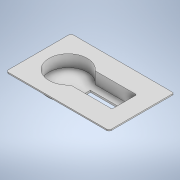
# Autodesk Inventor part: badge
Saved by Autodesk Inventor 2020 (Build 240168000, 168)
## iProperties
Created: 2019-12-22
Part Number: badge
Material: Generic
Document SubType Name: Modeling
Designer: user
Density: 1 g/cm^3
Appearance: Default
Author: user
## iProperties of the stored document _3DPrint.ipt
Created: 2019-12-23
Part Number: _3DPrint
Material: Generic
Document SubType Name: Modeling
Designer: user
Density: 1 g/cm^3
Appearance: Default
Author: user
Autodesk Inventor part; units mm, degrees
ref_plane "YZ Plane" through (0, 0, 0) normal (1, 0, 0) x (0, 1, 0)
ref_plane "XZ Plane" through (0, 0, 0) normal (0, 1, 0) x (-1, 0, 0)
ref_plane "XY Plane" through (0, 0, 0) normal (0, 0, 1) x (1, 0, 0)
sketch "Sketch1" plane through (0, 0, 0) normal (0, 1, 0) x (-1, 0, 0)
  circle A0 centre (-14.0224, -4.7987) radius 17
  line L0 (-61.8084, 4.4628) -> (-61.8084, -14.0372)
  line L1 (-59.8084, -16.0372) -> (-26.7776, -16.0372)
  line L2 (-26.7573, 6.4628) -> (-59.8084, 6.4628)
  arc A1 (-61.8084, -14.0372) -> (-59.8084, -16.0372) centre (-59.8084, -14.0372) ccw
  arc A2 (-59.8084, 6.4628) -> (-61.8084, 4.4628) centre (-59.8084, 4.4628) ccw
  line L3 (-28.2727, -0.5372) -> (-54.8084, -0.5372)
  line L4 (-54.8084, -0.5372) -> (-54.8084, -9.0372)
  line L5 (-54.8084, -9.0372) -> (-28.2727, -9.0372)
  line L6 (-28.2727, -9.0372) -> (-28.2727, -0.5372)
  line L7 (8.6213, 22.2028) -> (-72.9787, 22.2028)
  line L8 (-73.8987, -31.7772) -> (8.6213, -31.7772)
  line L9 (10.6213, -29.7772) -> (10.6213, 20.2028)
  line L10 (-74.9787, 20.2028) -> (-74.9787, 4.3773)
  line L11 (-74.9787, -30.6972) -> (-74.9787, -14.8717)
  arc A3 (-74.9787, -30.6972) -> (-73.8987, -31.7772) centre (-73.8987, -30.6972) ccw
  arc A4 (-72.9787, 22.2028) -> (-74.9787, 20.2028) centre (-72.9787, 20.2028) ccw
  arc A5 (10.6213, 20.2028) -> (8.6213, 22.2028) centre (8.6213, 20.2028) ccw
  arc A6 (8.6213, -31.7772) -> (10.6213, -29.7772) centre (8.6213, -29.7772) ccw
  line L12 (-74.9787, 4.3773) -> (-74.9787, -14.8717)
  circle A7 centre (-14.0224, -4.7987) radius 16
  line L13 (-27.4955, -15.0372) -> (-59.8084, -15.0372)
  line L14 (-60.8084, -14.0372) -> (-60.8084, 4.4628)
  arc A8 (-60.8084, -14.0372) -> (-59.8084, -15.0372) centre (-59.8084, -14.0372) ccw
  line L15 (-59.8084, 5.4628) -> (-27.576, 5.4628)
  arc A9 (-59.8084, 5.4628) -> (-60.8084, 4.4628) centre (-59.8084, 4.4628) ccw
  line L16 (-26.7776, -16.0372) -> (-25.4108, -16.0372)
  line L17 (-27.4955, -15.0372) -> (-26.3176, -15.0372)
  line L18 (-27.576, 5.4628) -> (-26.2984, 5.4628)
  line L19 (-26.7573, 6.4628) -> (-25.388, 6.4628)
  point P0 (0, 0)
  point P1 (-61.8084, -16.0372)
  dimension "d20" = 34
  dimension "d26" = 2
  dimension "d28" = 7
  dimension "d32" = 7
  dimension "d167" = 8.5
  dimension "d171" = 26.5357
  dimension "d177" = 85.6
  dimension "d229" = 32
  dimension "d230" = 1
  dimension "d231" = 1
  dimension "d232" = 1
  dimension "d233" = 1
  dimension "d234" = 1
  dimension "d235" = 1
  dimension "d241" = 53.98
  dimension "d242" = 22.74
  dimension "d243" = 22.74
  dimension "d248" = 62.786
  dimension "d249" = 6
  constraints: 40 end point, 23 point on circle, 16 tangent, 10 centre point, 6 horizontal, 6 parallel, 3 perpendicular, 3 point on line, 3 vertical, 2 equal radius
  measures "d20" diameter of A0
  measures "d26" radius of A1
  measures "d28" distance between parallel lines of L1 L5
  measures "d32" distance between parallel lines of L3 L2
  measures "d167" distance between parallel lines of L3 L5
  measures "d171" distance between parallel lines of L4 L6
  measures "d177" distance between parallel lines of L11 L9
  measures "d229" diameter of A7
  measures "d230" radial gap between concentric circles of A0 A7
  measures "d231" distance between parallel lines of L13 L1
  measures "d232" distance between parallel lines of L0 L14
  measures "d233" radius of A8
  measures "d234" distance between parallel lines of L2 L15
  measures "d235" radius of A9
  measures "d241" distance between parallel lines of L8 L7
  measures "d242" distance between parallel lines of L8 L5
  measures "d243" distance between parallel lines of L7 L3
  measures "d249" distance between parallel lines of L4 L14
extrude "Extrusion22" add sketch "Sketch1" along normal blind 1
extrude "Extrusion23" add sketch "Sketch1" against normal blind 10.5 contours A0 L16 A7 L19 | L19 A7 L18 A0 | A0 L15 A9 L14 A8 L13 L1 A1 L0 A2 L2 | A0 L13 L17 A7 L16 | L18 A7 L3 A0 | A0 L3 L4 L5 L13 A8 L14 A9 L15 | A7 L5 L6 L3 | A0 L5 A7 L17 L13 picked at (-18.1893, -4.791)
extrude "Extrusion24" cut sketch "Sketch1" against normal blind 9 contours L18 A7 L3 A0 | A0 L3 L4 L5 L13 A8 L14 A9 L15 | A7 L5 L6 L3 | A0 L5 A7 L17 L13 picked at (-18.1893, -4.791)
extrude "Extrusion25" add sketch "Sketch1" along normal blind 1 contours A0 L16 A7 L19 | L19 A7 L18 A0 | A0 L15 A9 L14 A8 L13 L1 A1 L0 A2 L2 | A0 L13 L17 A7 L16
sketch "Sketch24" plane through (0, 0, 0) normal (0, -1, 0) x (1, 0, 0)
  line L0 (30.3846, -19.8888) -> (77.1521, -19.8888) construction
  line L1 (77.1521, -19.8888) -> (77.1521, -30.5341) construction
  line L2 (77.1521, -30.5341) -> (30.3846, -30.5341) construction
  line L3 (30.3846, -30.5341) -> (30.3846, -19.8888) construction
  line L4 (40.073, -25.6301) -> (61.0048, -25.6301) construction
  line L5 (61.0048, -25.6301) -> (61.0048, -28.2616) construction
  line L6 (61.0048, -28.2616) -> (40.073, -28.2616) construction
  line L7 (40.073, -28.2616) -> (40.073, -25.6301) construction
  spline S0 degree 2 poles (31.7579, -23.0554) (31.4887, -23.0554) (31.0885, -22.9146) (30.9477, -22.7738) knots 0 0 0 1 2 2 2
  spline S1 degree 2 poles (30.9477, -22.7738) (30.7872, -22.6157) (30.6563, -22.1711) (30.6563, -21.8451) knots 0 0 0 1 2 2 2
  line L8 (30.6563, -21.8451) -> (30.6563, -19.9432)
  line L9 (30.6563, -19.9432) -> (31.0614, -19.9432)
  line L10 (31.0614, -19.9432) -> (31.0614, -21.8451)
  spline S2 degree 2 poles (31.0614, -21.8451) (31.0614, -22.0575) (31.1157, -22.344) (31.1923, -22.4601) knots 0 0 0 1 2 2 2
  spline S3 degree 2 poles (31.1923, -22.4601) (31.2738, -22.5836) (31.5554, -22.7096) (31.7579, -22.7096) knots 0 0 0 1 2 2 2
  spline S4 degree 2 poles (31.7579, -22.7096) (31.9481, -22.7096) (32.2445, -22.5836) (32.326, -22.4601) knots 0 0 0 1 2 2 2
  spline S5 degree 2 poles (32.326, -22.4601) (32.4026, -22.344) (32.4569, -22.06) (32.4569, -21.855) knots 0 0 0 1 2 2 2
  line L11 (32.4569, -21.855) -> (32.4569, -19.9432)
  line L12 (32.4569, -19.9432) -> (32.862, -19.9432)
  line L13 (32.862, -19.9432) -> (32.862, -21.8451)
  spline S6 degree 2 poles (32.862, -21.8451) (32.862, -22.1637) (32.7336, -22.6182) (32.5705, -22.7738) knots 0 0 0 1 2 2 2
  spline S7 degree 2 poles (32.5705, -22.7738) (32.4248, -22.9171) (32.0395, -23.0554) (31.7579, -23.0554) knots 0 0 0 1 2 2 2
  line L14 (35.6655, -22.9912) -> (35.1393, -22.9912)
  line L15 (35.1393, -22.9912) -> (34.0254, -21.5734)
  line L16 (34.0254, -21.5734) -> (33.8475, -21.7735)
  line L17 (33.8475, -21.7735) -> (33.8475, -22.9912)
  line L18 (33.8475, -22.9912) -> (33.4424, -22.9912)
  line L19 (33.4424, -22.9912) -> (33.4424, -19.9432)
  line L20 (33.4424, -19.9432) -> (33.8475, -19.9432)
  line L21 (33.8475, -19.9432) -> (33.8475, -21.3437)
  line L22 (33.8475, -21.3437) -> (35.0974, -19.9432)
  line L23 (35.0974, -19.9432) -> (35.5914, -19.9432)
  line L24 (35.5914, -19.9432) -> (34.3292, -21.3042)
  line L25 (34.3292, -21.3042) -> (35.6655, -22.9912)
  line L26 (38.2787, -22.9912) -> (37.0981, -22.9912)
  line L27 (37.0981, -22.9912) -> (37.0981, -22.68)
  line L28 (37.0981, -22.68) -> (37.4859, -22.68)
  line L29 (37.4859, -22.68) -> (37.4859, -20.2544)
  line L30 (37.4859, -20.2544) -> (37.0981, -20.2544)
  line L31 (37.0981, -20.2544) -> (37.0981, -19.9432)
  line L32 (37.0981, -19.9432) -> (38.2787, -19.9432)
  line L33 (38.2787, -19.9432) -> (38.2787, -20.2544)
  line L34 (38.2787, -20.2544) -> (37.8909, -20.2544)
  line L35 (37.8909, -20.2544) -> (37.8909, -22.68)
  line L36 (37.8909, -22.68) -> (38.2787, -22.68)
  line L37 (38.2787, -22.68) -> (38.2787, -22.9912)
  line L38 (40.9612, -22.9912) -> (40.5067, -22.9912)
  line L39 (40.5067, -22.9912) -> (39.1581, -20.3631)
  line L40 (39.1581, -20.3631) -> (39.1581, -22.9912)
  line L41 (39.1581, -22.9912) -> (38.7802, -22.9912)
  line L42 (38.7802, -22.9912) -> (38.7802, -19.9432)
  line L43 (38.7802, -19.9432) -> (39.3557, -19.9432)
  line L44 (39.3557, -19.9432) -> (40.5833, -22.3564)
  line L45 (40.5833, -22.3564) -> (40.5833, -19.9432)
  line L46 (40.5833, -19.9432) -> (40.9612, -19.9432)
  line L47 (40.9612, -19.9432) -> (40.9612, -22.9912)
  spline S8 degree 2 poles (42.7692, -23.0455) (42.4728, -23.0455) (41.9714, -22.8455) (41.7886, -22.6454) knots 0 0 0 1 2 2 2
  spline S9 degree 2 poles (41.7886, -22.6454) (41.6059, -22.4478) (41.4058, -21.855) (41.4058, -21.4697) knots 0 0 0 1 2 2 2
  spline S10 degree 2 poles (41.4058, -21.4697) (41.4058, -21.0868) (41.6009, -20.5187) (41.7862, -20.3087) knots 0 0 0 1 2 2 2
  spline S11 degree 2 poles (41.7862, -20.3087) (41.9689, -20.1037) (42.4679, -19.8888) (42.7766, -19.8888) knots 0 0 0 1 2 2 2
  spline S12 degree 2 poles (42.7766, -19.8888) (42.9298, -19.8888) (43.199, -19.9333) (43.3126, -19.9679) knots 0 0 0 1 2 2 2
  spline S13 degree 2 poles (43.3126, -19.9679) (43.4114, -20) (43.6164, -20.0914) (43.7177, -20.1457) knots 0 0 0 1 2 2 2
  line L48 (43.7177, -20.1457) -> (43.7177, -20.6348)
  line L49 (43.7177, -20.6348) -> (43.6856, -20.6348)
  spline S14 degree 2 poles (43.6856, -20.6348) (43.6313, -20.5854) (43.4633, -20.4471) (43.3423, -20.3804) knots 0 0 0 1 2 2 2
  spline S15 degree 2 poles (43.3423, -20.3804) (43.2262, -20.3162) (42.952, -20.2346) (42.7742, -20.2346) knots 0 0 0 1 2 2 2
  spline S16 degree 2 poles (42.7742, -20.2346) (42.579, -20.2346) (42.2308, -20.3952) (42.0999, -20.5483) knots 0 0 0 1 2 2 2
  spline S17 degree 2 poles (42.0999, -20.5483) (41.9714, -20.704) (41.8282, -21.1757) (41.8282, -21.4697) knots 0 0 0 1 2 2 2
  spline S18 degree 2 poles (41.8282, -21.4697) (41.8282, -21.7833) (41.9788, -22.2354) (42.1097, -22.391) knots 0 0 0 1 2 2 2
  spline S19 degree 2 poles (42.1097, -22.391) (42.2382, -22.5416) (42.5815, -22.6948) (42.7742, -22.6948) knots 0 0 0 1 2 2 2
  spline S20 degree 2 poles (42.7742, -22.6948) (42.9495, -22.6948) (43.2484, -22.6083) (43.3645, -22.5441) knots 0 0 0 1 2 2 2
  spline S21 degree 2 poles (43.3645, -22.5441) (43.4757, -22.4799) (43.6411, -22.3465) (43.6881, -22.2996) knots 0 0 0 1 2 2 2
  line L50 (43.6881, -22.2996) -> (43.7177, -22.2996)
  line L51 (43.7177, -22.2996) -> (43.7177, -22.7837)
  spline S22 degree 2 poles (43.7177, -22.7837) (43.6164, -22.8306) (43.4386, -22.9171) (43.3126, -22.9566) knots 0 0 0 1 2 2 2
  spline S23 degree 2 poles (43.3126, -22.9566) (43.1793, -23.0011) (42.952, -23.0455) (42.7692, -23.0455) knots 0 0 0 1 2 2 2
  line L52 (45.1577, -22.9912) -> (43.9771, -22.9912)
  line L53 (43.9771, -22.9912) -> (43.9771, -22.68)
  line L54 (43.9771, -22.68) -> (44.3649, -22.68)
  line L55 (44.3649, -22.68) -> (44.3649, -20.2544)
  line L56 (44.3649, -20.2544) -> (43.9771, -20.2544)
  line L57 (43.9771, -20.2544) -> (43.9771, -19.9432)
  line L58 (43.9771, -19.9432) -> (45.1577, -19.9432)
  line L59 (45.1577, -19.9432) -> (45.1577, -20.2544)
  line L60 (45.1577, -20.2544) -> (44.7699, -20.2544)
  line L61 (44.7699, -20.2544) -> (44.7699, -22.68)
  line L62 (44.7699, -22.68) -> (45.1577, -22.68)
  line L63 (45.1577, -22.68) -> (45.1577, -22.9912)
  spline S24 degree 2 poles (48.0625, -21.4697) (48.0625, -21.8871) (47.7241, -22.5589) (47.44, -22.7467) knots 0 0 0 1 2 2 2
  spline S25 degree 2 poles (47.44, -22.7467) (47.2078, -22.8924) (46.7311, -22.9912) (46.3606, -22.9912) knots 0 0 0 1 2 2 2
  line L64 (46.3606, -22.9912) -> (45.6591, -22.9912)
  line L65 (45.6591, -22.9912) -> (45.6591, -19.9432)
  line L66 (45.6591, -19.9432) -> (46.3532, -19.9432)
  spline S26 degree 2 poles (46.3532, -19.9432) (46.783, -19.9432) (47.2721, -20.0716) (47.445, -20.1852) knots 0 0 0 1 2 2 2
  spline S27 degree 2 poles (47.445, -20.1852) (47.7389, -20.3804) (48.0625, -21.0251) (48.0625, -21.4697) knots 0 0 0 1 2 2 2
  spline S28 degree 2 poles (47.6401, -21.4647) (47.6401, -21.114) (47.4079, -20.6175) (47.1782, -20.4767) knots 0 0 0 1 2 2 2
  spline S29 degree 2 poles (47.1782, -20.4767) (47.0152, -20.3804) (46.6472, -20.2939) (46.373, -20.2939) knots 0 0 0 1 2 2 2
  line L67 (46.373, -20.2939) -> (46.0642, -20.2939)
  line L68 (46.0642, -20.2939) -> (46.0642, -22.6404)
  line L69 (46.0642, -22.6404) -> (46.373, -22.6404)
  spline S30 degree 2 poles (46.373, -22.6404) (46.6422, -22.6404) (47.0498, -22.554) (47.2153, -22.4379) knots 0 0 0 1 2 2 2
  spline S31 degree 2 poles (47.2153, -22.4379) (47.4277, -22.2946) (47.6401, -21.8204) (47.6401, -21.4647) knots 0 0 0 1 2 2 2
  line L70 (48.5021, -22.9912) -> (48.5021, -19.9432)
  line L71 (48.5021, -19.9432) -> (50.409, -19.9432)
  line L72 (50.409, -19.9432) -> (50.409, -20.3038)
  line L73 (50.409, -20.3038) -> (48.9072, -20.3038)
  line L74 (48.9072, -20.3038) -> (48.9072, -21.1387)
  line L75 (48.9072, -21.1387) -> (50.3077, -21.1387)
  line L76 (50.3077, -21.1387) -> (50.3077, -21.4993)
  line L77 (50.3077, -21.4993) -> (48.9072, -21.4993)
  line L78 (48.9072, -21.4993) -> (48.9072, -22.6306)
  line L79 (48.9072, -22.6306) -> (50.409, -22.6306)
  line L80 (50.409, -22.6306) -> (50.409, -22.9912)
  line L81 (50.409, -22.9912) -> (48.5021, -22.9912)
  line L82 (53.0346, -22.9912) -> (52.5801, -22.9912)
  line L83 (52.5801, -22.9912) -> (51.2315, -20.3631)
  line L84 (51.2315, -20.3631) -> (51.2315, -22.9912)
  line L85 (51.2315, -22.9912) -> (50.8536, -22.9912)
  line L86 (50.8536, -22.9912) -> (50.8536, -19.9432)
  line L87 (50.8536, -19.9432) -> (51.4291, -19.9432)
  line L88 (51.4291, -19.9432) -> (52.6567, -22.3564)
  line L89 (52.6567, -22.3564) -> (52.6567, -19.9432)
  line L90 (52.6567, -19.9432) -> (53.0346, -19.9432)
  line L91 (53.0346, -19.9432) -> (53.0346, -22.9912)
  line L92 (54.3635, -22.9912) -> (54.3635, -20.3038)
  line L93 (54.3635, -20.3038) -> (53.3409, -20.3038)
  line L94 (53.3409, -20.3038) -> (53.3409, -19.9432)
  line L95 (53.3409, -19.9432) -> (55.7912, -19.9432)
  line L96 (55.7912, -19.9432) -> (55.7912, -20.3038)
  line L97 (55.7912, -20.3038) -> (54.7686, -20.3038)
  line L98 (54.7686, -20.3038) -> (54.7686, -22.9912)
  line L99 (54.7686, -22.9912) -> (54.3635, -22.9912)
  line L100 (59.59, -22.9912) -> (59.1356, -22.9912)
  line L101 (59.1356, -22.9912) -> (57.7869, -20.3631)
  line L102 (57.7869, -20.3631) -> (57.7869, -22.9912)
  line L103 (57.7869, -22.9912) -> (57.409, -22.9912)
  line L104 (57.409, -22.9912) -> (57.409, -19.9432)
  line L105 (57.409, -19.9432) -> (57.9845, -19.9432)
  line L106 (57.9845, -19.9432) -> (59.2121, -22.3564)
  line L107 (59.2121, -22.3564) -> (59.2121, -19.9432)
  line L108 (59.2121, -19.9432) -> (59.59, -19.9432)
  line L109 (59.59, -19.9432) -> (59.59, -22.9912)
  spline S32 degree 2 poles (61.2721, -23.0554) (61.0029, -23.0554) (60.6027, -22.9146) (60.462, -22.7738) knots 0 0 0 1 2 2 2
  spline S33 degree 2 poles (60.462, -22.7738) (60.3014, -22.6157) (60.1705, -22.1711) (60.1705, -21.8451) knots 0 0 0 1 2 2 2
  line L110 (60.1705, -21.8451) -> (60.1705, -19.9432)
  line L111 (60.1705, -19.9432) -> (60.5756, -19.9432)
  line L112 (60.5756, -19.9432) -> (60.5756, -21.8451)
  spline S34 degree 2 poles (60.5756, -21.8451) (60.5756, -22.0575) (60.6299, -22.344) (60.7065, -22.4601) knots 0 0 0 1 2 2 2
  spline S35 degree 2 poles (60.7065, -22.4601) (60.788, -22.5836) (61.0696, -22.7096) (61.2721, -22.7096) knots 0 0 0 1 2 2 2
  spline S36 degree 2 poles (61.2721, -22.7096) (61.4623, -22.7096) (61.7587, -22.5836) (61.8402, -22.4601) knots 0 0 0 1 2 2 2
  spline S37 degree 2 poles (61.8402, -22.4601) (61.9168, -22.344) (61.9711, -22.06) (61.9711, -21.855) knots 0 0 0 1 2 2 2
  line L113 (61.9711, -21.855) -> (61.9711, -19.9432)
  line L114 (61.9711, -19.9432) -> (62.3762, -19.9432)
  line L115 (62.3762, -19.9432) -> (62.3762, -21.8451)
  spline S38 degree 2 poles (62.3762, -21.8451) (62.3762, -22.1637) (62.2478, -22.6182) (62.0848, -22.7738) knots 0 0 0 1 2 2 2
  spline S39 degree 2 poles (62.0848, -22.7738) (61.939, -22.9171) (61.5537, -23.0554) (61.2721, -23.0554) knots 0 0 0 1 2 2 2
  line L116 (65.5699, -22.9912) -> (65.1649, -22.9912)
  line L117 (65.1649, -22.9912) -> (65.1649, -20.3656)
  line L118 (65.1649, -20.3656) -> (64.3695, -22.1514)
  line L119 (64.3695, -22.1514) -> (64.1225, -22.1514)
  line L120 (64.1225, -22.1514) -> (63.3346, -20.3656)
  line L121 (63.3346, -20.3656) -> (63.3346, -22.9912)
  line L122 (63.3346, -22.9912) -> (62.9567, -22.9912)
  line L123 (62.9567, -22.9912) -> (62.9567, -19.9432)
  line L124 (62.9567, -19.9432) -> (63.51, -19.9432)
  line L125 (63.51, -19.9432) -> (64.2707, -21.6401)
  line L126 (64.2707, -21.6401) -> (65.0068, -19.9432)
  line L127 (65.0068, -19.9432) -> (65.5699, -19.9432)
  line L128 (65.5699, -19.9432) -> (65.5699, -22.9912)
  spline S40 degree 2 poles (68.2549, -22.0551) (68.2549, -22.2823) (68.082, -22.6306) (67.9387, -22.7442) knots 0 0 0 1 2 2 2
  spline S41 degree 2 poles (67.9387, -22.7442) (67.7658, -22.8776) (67.3731, -22.9912) (67.0618, -22.9912) knots 0 0 0 1 2 2 2
  line L129 (67.0618, -22.9912) -> (66.1875, -22.9912)
  line L130 (66.1875, -22.9912) -> (66.1875, -19.9432)
  line L131 (66.1875, -19.9432) -> (66.9951, -19.9432)
  spline S42 degree 2 poles (66.9951, -19.9432) (67.3212, -19.9432) (67.6472, -19.9852) (67.7954, -20.0667) knots 0 0 0 1 2 2 2
  spline S43 degree 2 poles (67.7954, -20.0667) (67.9609, -20.1531) (68.1116, -20.4372) (68.1116, -20.6299) knots 0 0 0 1 2 2 2
  spline S44 degree 2 poles (68.1116, -20.6299) (68.1116, -20.8447) (67.8844, -21.1856) (67.6843, -21.2819) knots 0 0 0 1 2 2 2
  line L132 (67.6843, -21.2819) -> (67.6843, -21.2968)
  spline S45 degree 2 poles (67.6843, -21.2968) (67.956, -21.3709) (68.2549, -21.7636) (68.2549, -22.0551) knots 0 0 0 1 2 2 2
  spline S46 degree 2 poles (67.8325, -22.0723) (67.8325, -21.8994) (67.7337, -21.6771) (67.5855, -21.5981) knots 0 0 0 1 2 2 2
  spline S47 degree 2 poles (67.5855, -21.5981) (67.4892, -21.5487) (67.2619, -21.5191) (67.052, -21.5191) knots 0 0 0 1 2 2 2
  line L133 (67.052, -21.5191) -> (66.5925, -21.5191)
  line L134 (66.5925, -21.5191) -> (66.5925, -22.6454)
  line L135 (66.5925, -22.6454) -> (66.921, -22.6454)
  spline S48 degree 2 poles (66.921, -22.6454) (67.1878, -22.6454) (67.4941, -22.596) (67.6127, -22.5169) knots 0 0 0 1 2 2 2
  spline S49 degree 2 poles (67.6127, -22.5169) (67.7263, -22.4354) (67.8325, -22.2329) (67.8325, -22.0723) knots 0 0 0 1 2 2 2
  spline S50 degree 2 poles (67.6892, -20.6867) (67.6892, -20.578) (67.6151, -20.415) (67.5336, -20.368) knots 0 0 0 1 2 2 2
  spline S51 degree 2 poles (67.5336, -20.368) (67.4348, -20.3137) (67.1952, -20.289) (66.9803, -20.289) knots 0 0 0 1 2 2 2
  line L136 (66.9803, -20.289) -> (66.5925, -20.289)
  line L137 (66.5925, -20.289) -> (66.5925, -21.1807)
  line L138 (66.5925, -21.1807) -> (67.052, -21.1807)
  spline S52 degree 2 poles (67.052, -21.1807) (67.2421, -21.1807) (67.4225, -21.1411) (67.5188, -21.0794) knots 0 0 0 1 2 2 2
  spline S53 degree 2 poles (67.5188, -21.0794) (67.6127, -21.0201) (67.6892, -20.8299) (67.6892, -20.6867) knots 0 0 0 1 2 2 2
  line L139 (68.6575, -22.9912) -> (68.6575, -19.9432)
  line L140 (68.6575, -19.9432) -> (70.5643, -19.9432)
  line L141 (70.5643, -19.9432) -> (70.5643, -20.3038)
  line L142 (70.5643, -20.3038) -> (69.0626, -20.3038)
  line L143 (69.0626, -20.3038) -> (69.0626, -21.1387)
  line L144 (69.0626, -21.1387) -> (70.4631, -21.1387)
  line L145 (70.4631, -21.1387) -> (70.4631, -21.4993)
  line L146 (70.4631, -21.4993) -> (69.0626, -21.4993)
  line L147 (69.0626, -21.4993) -> (69.0626, -22.6306)
  line L148 (69.0626, -22.6306) -> (70.5643, -22.6306)
  line L149 (70.5643, -22.6306) -> (70.5643, -22.9912)
  line L150 (70.5643, -22.9912) -> (68.6575, -22.9912)
  line L151 (73.3678, -22.9912) -> (72.8417, -22.9912)
  line L152 (72.8417, -22.9912) -> (71.8784, -21.7784)
  line L153 (71.8784, -21.7784) -> (71.414, -21.7784)
  line L154 (71.414, -21.7784) -> (71.414, -22.9912)
  line L155 (71.414, -22.9912) -> (71.0089, -22.9912)
  line L156 (71.0089, -22.9912) -> (71.0089, -19.9432)
  line L157 (71.0089, -19.9432) -> (71.7944, -19.9432)
  spline S54 degree 2 poles (71.7944, -19.9432) (72.0562, -19.9432) (72.4094, -20) (72.57, -20.1037) knots 0 0 0 1 2 2 2
  spline S55 degree 2 poles (72.57, -20.1037) (72.7305, -20.2075) (72.9158, -20.5311) (72.9158, -20.7706) knots 0 0 0 1 2 2 2
  spline S56 degree 2 poles (72.9158, -20.7706) (72.9158, -21.1041) (72.5749, -21.5561) (72.2835, -21.6648) knots 0 0 0 1 2 2 2
  line L158 (72.2835, -21.6648) -> (73.3678, -22.9912)
  spline S57 degree 2 poles (72.4934, -20.8028) (72.4934, -20.6694) (72.3995, -20.4644) (72.3007, -20.3977) knots 0 0 0 1 2 2 2
  spline S58 degree 2 poles (72.3007, -20.3977) (72.2143, -20.3409) (71.9846, -20.2939) (71.8166, -20.2939) knots 0 0 0 1 2 2 2
  line L159 (71.8166, -20.2939) -> (71.414, -20.2939)
  line L160 (71.414, -20.2939) -> (71.414, -21.44)
  line L161 (71.414, -21.44) -> (71.7697, -21.44)
  spline S59 degree 2 poles (71.7697, -21.44) (71.9451, -21.44) (72.2242, -21.3783) (72.3205, -21.2819) knots 0 0 0 1 2 2 2
  spline S60 degree 2 poles (72.3205, -21.2819) (72.4094, -21.198) (72.4934, -20.9608) (72.4934, -20.8028) knots 0 0 0 1 2 2 2
  spline S61 degree 2 poles (42.1923, -27.2233) (42.1923, -28.0433) (41.7155, -28.8115) (41.2191, -28.8115) knots 0 0 0 1 2 2 2
  spline S62 degree 2 poles (41.2191, -28.8115) (40.7152, -28.8115) (40.2434, -28.0285) (40.2434, -27.2258) knots 0 0 0 1 2 2 2
  spline S63 degree 2 poles (40.2434, -27.2258) (40.2434, -26.4008) (40.7201, -25.6375) (41.2191, -25.6375) knots 0 0 0 1 2 2 2
  spline S64 degree 2 poles (41.2191, -25.6375) (41.7205, -25.6375) (42.1923, -26.4279) (42.1923, -27.2233) knots 0 0 0 1 2 2 2
  spline S65 degree 2 poles (41.6686, -28.152) (41.7279, -28.0013) (41.7773, -27.537) (41.7773, -27.2233) knots 0 0 0 1 2 2 2
  spline S66 degree 2 poles (41.7773, -27.2233) (41.7773, -26.9096) (41.7279, -26.4477) (41.6661, -26.2921) knots 0 0 0 1 2 2 2
  spline S67 degree 2 poles (41.6661, -26.2921) (41.6044, -26.1365) (41.3895, -25.9759) (41.2191, -25.9759) knots 0 0 0 1 2 2 2
  spline S68 degree 2 poles (41.2191, -25.9759) (41.0486, -25.9759) (40.8288, -26.1365) (40.7646, -26.297) knots 0 0 0 1 2 2 2
  spline S69 degree 2 poles (40.7646, -26.297) (40.7028, -26.4526) (40.6584, -26.9269) (40.6584, -27.2258) knots 0 0 0 1 2 2 2
  spline S70 degree 2 poles (40.6584, -27.2258) (40.6584, -27.5469) (40.6979, -27.9766) (40.7621, -28.1446) knots 0 0 0 1 2 2 2
  spline S71 degree 2 poles (40.7621, -28.1446) (40.8214, -28.3027) (41.0412, -28.4731) (41.2191, -28.4731) knots 0 0 0 1 2 2 2
  spline S72 degree 2 poles (41.2191, -28.4731) (41.387, -28.4731) (41.6069, -28.3126) (41.6686, -28.152) knots 0 0 0 1 2 2 2
  line L162 (44.3091, -28.7473) -> (42.8221, -28.7473)
  line L163 (42.8221, -28.7473) -> (42.8221, -28.4361)
  line L164 (42.8221, -28.4361) -> (43.3754, -28.4361)
  line L165 (43.3754, -28.4361) -> (43.3754, -26.3934)
  line L166 (43.3754, -26.3934) -> (42.8221, -26.3934)
  line L167 (42.8221, -26.3934) -> (42.8221, -26.1143)
  spline S73 degree 2 poles (42.8221, -26.1143) (43.1358, -26.1143) (43.4322, -25.9364) (43.452, -25.6894) knots 0 0 0 1 2 2 2
  line L168 (43.452, -25.6894) -> (43.7681, -25.6894)
  line L169 (43.7681, -25.6894) -> (43.7681, -28.4361)
  line L170 (43.7681, -28.4361) -> (44.3091, -28.4361)
  line L171 (44.3091, -28.4361) -> (44.3091, -28.7473)
  line L172 (46.8309, -27.7) -> (46.4679, -27.7)
  line L173 (46.4679, -27.7) -> (46.4679, -28.7473)
  line L174 (46.4679, -28.7473) -> (46.0751, -28.7473)
  line L175 (46.0751, -28.7473) -> (46.0751, -27.7)
  line L176 (46.0751, -27.7) -> (44.729, -27.7)
  line L177 (44.729, -27.7) -> (44.729, -27.2702)
  line L178 (44.729, -27.2702) -> (46.0924, -25.6993)
  line L179 (46.0924, -25.6993) -> (46.4679, -25.6993)
  line L180 (46.4679, -25.6993) -> (46.4679, -27.3715)
  line L181 (46.4679, -27.3715) -> (46.8309, -27.3715)
  line L182 (46.8309, -27.3715) -> (46.8309, -27.7)
  line L183 (46.0751, -27.3715) -> (46.0751, -26.1809)
  line L184 (46.0751, -26.1809) -> (45.0501, -27.3715)
  line L185 (45.0501, -27.3715) -> (46.0751, -27.3715)
  spline S74 degree 2 poles (48.0783, -28.8165) (47.8511, -28.8165) (47.4781, -28.6806) (47.3472, -28.5546) knots 0 0 0 1 2 2 2
  spline S75 degree 2 poles (47.3472, -28.5546) (47.2187, -28.4311) (47.0854, -28.0952) (47.0854, -27.905) knots 0 0 0 1 2 2 2
  spline S76 degree 2 poles (47.0854, -27.905) (47.0854, -27.658) (47.3497, -27.2431) (47.6016, -27.1196) knots 0 0 0 1 2 2 2
  line L186 (47.6016, -27.1196) -> (47.6016, -27.1072)
  spline S77 degree 2 poles (47.6016, -27.1072) (47.3768, -26.9763) (47.1595, -26.6651) (47.1595, -26.4329) knots 0 0 0 1 2 2 2
  spline S78 degree 2 poles (47.1595, -26.4329) (47.1595, -26.0896) (47.6782, -25.6301) (48.0783, -25.6301) knots 0 0 0 1 2 2 2
  spline S79 degree 2 poles (48.0783, -25.6301) (48.4933, -25.6301) (48.9947, -26.0649) (48.9947, -26.4057) knots 0 0 0 1 2 2 2
  spline S80 degree 2 poles (48.9947, -26.4057) (48.9947, -26.6107) (48.7551, -27.0109) (48.5303, -27.1245) knots 0 0 0 1 2 2 2
  line L187 (48.5303, -27.1245) -> (48.5303, -27.1368)
  spline S81 degree 2 poles (48.5303, -27.1368) (48.7971, -27.2603) (49.0713, -27.616) (49.0713, -27.8976) knots 0 0 0 1 2 2 2
  spline S82 degree 2 poles (49.0713, -27.8976) (49.0713, -28.2879) (48.5032, -28.8165) (48.0783, -28.8165) knots 0 0 0 1 2 2 2
  spline S83 degree 2 poles (48.6514, -27.9371) (48.6514, -27.7494) (48.5032, -27.5271) (48.2932, -27.4135) knots 0 0 0 1 2 2 2
  spline S84 degree 2 poles (48.2932, -27.4135) (48.224, -27.374) (47.9919, -27.2826) (47.8461, -27.2233) knots 0 0 0 1 2 2 2
  spline S85 degree 2 poles (47.8461, -27.2233) (47.6782, -27.3344) (47.4979, -27.6654) (47.4979, -27.8754) knots 0 0 0 1 2 2 2
  spline S86 degree 2 poles (47.4979, -27.8754) (47.4979, -28.152) (47.8313, -28.5126) (48.0832, -28.5126) knots 0 0 0 1 2 2 2
  spline S87 degree 2 poles (48.0832, -28.5126) (48.3401, -28.5126) (48.6514, -28.2039) (48.6514, -27.9371) knots 0 0 0 1 2 2 2
  spline S88 degree 2 poles (48.5945, -26.4107) (48.5945, -26.2056) (48.3204, -25.9315) (48.0758, -25.9315) knots 0 0 0 1 2 2 2
  spline S89 degree 2 poles (48.0758, -25.9315) (47.8535, -25.9315) (47.5695, -26.176) (47.5695, -26.386) knots 0 0 0 1 2 2 2
  spline S90 degree 2 poles (47.5695, -26.386) (47.5695, -26.5366) (47.7152, -26.7466) (47.8609, -26.8306) knots 0 0 0 1 2 2 2
  spline S91 degree 2 poles (47.8609, -26.8306) (47.9227, -26.8651) (48.1845, -26.9862) (48.2907, -27.0208) knots 0 0 0 1 2 2 2
  spline S92 degree 2 poles (48.2907, -27.0208) (48.4686, -26.8849) (48.5945, -26.5959) (48.5945, -26.4107) knots 0 0 0 1 2 2 2
  spline S93 degree 2 poles (50.2667, -25.9883) (50.1556, -25.9883) (49.9358, -26.0426) (49.8295, -26.0846) knots 0 0 0 1 2 2 2
  spline S94 degree 2 poles (49.8295, -26.0846) (49.7307, -26.1266) (49.585, -26.2155) (49.5282, -26.255) knots 0 0 0 1 2 2 2
  line L188 (49.5282, -26.255) -> (49.5035, -26.255)
  line L189 (49.5035, -26.255) -> (49.5035, -25.8228)
  spline S95 degree 2 poles (49.5035, -25.8228) (49.6369, -25.7512) (50.0938, -25.6351) (50.2989, -25.6351) knots 0 0 0 1 2 2 2
  spline S96 degree 2 poles (50.2989, -25.6351) (50.5063, -25.6351) (50.8151, -25.7191) (50.9411, -25.808) knots 0 0 0 1 2 2 2
  spline S97 degree 2 poles (50.9411, -25.808) (51.0744, -25.9043) (51.2128, -26.1834) (51.2128, -26.3711) knots 0 0 0 1 2 2 2
  spline S98 degree 2 poles (51.2128, -26.3711) (51.2128, -26.6231) (50.8818, -27.0035) (50.6496, -27.0529) knots 0 0 0 1 2 2 2
  line L190 (50.6496, -27.0529) -> (50.6496, -27.0825)
  spline S99 degree 2 poles (50.6496, -27.0825) (50.7459, -27.1023) (50.9658, -27.1912) (51.0596, -27.2801) knots 0 0 0 1 2 2 2
  spline S100 degree 2 poles (51.0596, -27.2801) (51.1535, -27.3666) (51.272, -27.6432) (51.272, -27.8433) knots 0 0 0 1 2 2 2
  spline S101 degree 2 poles (51.272, -27.8433) (51.272, -28.0483) (51.1312, -28.3965) (51.0028, -28.5299) knots 0 0 0 1 2 2 2
  spline S102 degree 2 poles (51.0028, -28.5299) (50.8694, -28.6683) (50.4915, -28.8115) (50.2519, -28.8115) knots 0 0 0 1 2 2 2
  spline S103 degree 2 poles (50.2519, -28.8115) (50.0222, -28.8115) (49.5727, -28.7004) (49.4195, -28.6238) knots 0 0 0 1 2 2 2
  line L191 (49.4195, -28.6238) -> (49.4195, -28.1915)
  line L192 (49.4195, -28.1915) -> (49.4492, -28.1915)
  spline S104 degree 2 poles (49.4492, -28.1915) (49.5776, -28.2854) (50.0123, -28.4583) (50.2272, -28.4583) knots 0 0 0 1 2 2 2
  spline S105 degree 2 poles (50.2272, -28.4583) (50.3532, -28.4583) (50.6051, -28.3793) (50.6891, -28.2879) knots 0 0 0 1 2 2 2
  spline S106 degree 2 poles (50.6891, -28.2879) (50.7706, -28.1965) (50.8571, -27.9791) (50.8571, -27.8136) knots 0 0 0 1 2 2 2
  spline S107 degree 2 poles (50.8571, -27.8136) (50.8571, -27.6481) (50.7607, -27.4332) (50.6743, -27.3715) knots 0 0 0 1 2 2 2
  spline S108 degree 2 poles (50.6743, -27.3715) (50.5878, -27.3097) (50.3532, -27.2628) (50.2149, -27.2628) knots 0 0 0 1 2 2 2
  line L193 (50.2149, -27.2628) -> (50.042, -27.2628)
  line L194 (50.042, -27.2628) -> (50.042, -26.9244)
  line L195 (50.042, -26.9244) -> (50.1778, -26.9244)
  spline S109 degree 2 poles (50.1778, -26.9244) (50.452, -26.9244) (50.7978, -26.6626) (50.7978, -26.4131) knots 0 0 0 1 2 2 2
  spline S110 degree 2 poles (50.7978, -26.4131) (50.7978, -26.297) (50.7089, -26.1315) (50.6372, -26.0821) knots 0 0 0 1 2 2 2
  spline S111 degree 2 poles (50.6372, -26.0821) (50.5607, -26.0303) (50.373, -25.9883) (50.2667, -25.9883) knots 0 0 0 1 2 2 2
  spline S112 degree 2 poles (53.6581, -27.7593) (53.6581, -27.9939) (53.5025, -28.3916) (53.3716, -28.525) knots 0 0 0 1 2 2 2
  spline S113 degree 2 poles (53.3716, -28.525) (53.2357, -28.6658) (52.8948, -28.8115) (52.6898, -28.8115) knots 0 0 0 1 2 2 2
  spline S114 degree 2 poles (52.6898, -28.8115) (52.4848, -28.8115) (52.1464, -28.6732) (52.018, -28.5349) knots 0 0 0 1 2 2 2
  spline S115 degree 2 poles (52.018, -28.5349) (51.8599, -28.3694) (51.6821, -27.8136) (51.6821, -27.4085) knots 0 0 0 1 2 2 2
  spline S116 degree 2 poles (51.6821, -27.4085) (51.6821, -27.0109) (51.8451, -26.3711) (52.0155, -26.134) knots 0 0 0 1 2 2 2
  spline S117 degree 2 poles (52.0155, -26.134) (52.181, -25.9018) (52.7046, -25.6425) (53.048, -25.6425) knots 0 0 0 1 2 2 2
  spline S118 degree 2 poles (53.048, -25.6425) (53.1493, -25.6425) (53.3271, -25.6622) (53.3938, -25.6845) knots 0 0 0 1 2 2 2
  line L196 (53.3938, -25.6845) -> (53.3938, -26.0772)
  line L197 (53.3938, -26.0772) -> (53.3765, -26.0772)
  spline S119 degree 2 poles (53.3765, -26.0772) (53.3197, -26.0476) (53.1122, -25.9957) (52.9936, -25.9957) knots 0 0 0 1 2 2 2
  spline S120 degree 2 poles (52.9936, -25.9957) (52.6133, -25.9957) (52.1464, -26.5095) (52.102, -27.0133) knots 0 0 0 1 2 2 2
  spline S121 degree 2 poles (52.102, -27.0133) (52.2477, -26.9121) (52.554, -26.8009) (52.7368, -26.8009) knots 0 0 0 1 2 2 2
  spline S122 degree 2 poles (52.7368, -26.8009) (52.9146, -26.8009) (53.1814, -26.8725) (53.3271, -26.9812) knots 0 0 0 1 2 2 2
  spline S123 degree 2 poles (53.3271, -26.9812) (53.4951, -27.1072) (53.6581, -27.4975) (53.6581, -27.7593) knots 0 0 0 1 2 2 2
  spline S124 degree 2 poles (53.2431, -27.7766) (53.2431, -27.5889) (53.1443, -27.3344) (53.0356, -27.2455) knots 0 0 0 1 2 2 2
  spline S125 degree 2 poles (53.0356, -27.2455) (52.9541, -27.1813) (52.7516, -27.1393) (52.6454, -27.1393) knots 0 0 0 1 2 2 2
  spline S126 degree 2 poles (52.6454, -27.1393) (52.5021, -27.1393) (52.2329, -27.2258) (52.102, -27.3073) knots 0 0 0 1 2 2 2
  spline S127 degree 2 poles (52.102, -27.3073) (52.0995, -27.3517) (52.0946, -27.4357) (52.0946, -27.4999) knots 0 0 0 1 2 2 2
  spline S128 degree 2 poles (52.0946, -27.4999) (52.0946, -27.8161) (52.2181, -28.2039) (52.3119, -28.3052) knots 0 0 0 1 2 2 2
  spline S129 degree 2 poles (52.3119, -28.3052) (52.3984, -28.4015) (52.5861, -28.4781) (52.6923, -28.4781) knots 0 0 0 1 2 2 2
  spline S130 degree 2 poles (52.6923, -28.4781) (52.9393, -28.4781) (53.2431, -28.1273) (53.2431, -27.7766) knots 0 0 0 1 2 2 2
  spline S131 degree 2 poles (55.9453, -27.7593) (55.9453, -27.9939) (55.7897, -28.3916) (55.6588, -28.525) knots 0 0 0 1 2 2 2
  spline S132 degree 2 poles (55.6588, -28.525) (55.5229, -28.6658) (55.1821, -28.8115) (54.9771, -28.8115) knots 0 0 0 1 2 2 2
  spline S133 degree 2 poles (54.9771, -28.8115) (54.7721, -28.8115) (54.4337, -28.6732) (54.3052, -28.5349) knots 0 0 0 1 2 2 2
  spline S134 degree 2 poles (54.3052, -28.5349) (54.1471, -28.3694) (53.9693, -27.8136) (53.9693, -27.4085) knots 0 0 0 1 2 2 2
  spline S135 degree 2 poles (53.9693, -27.4085) (53.9693, -27.0109) (54.1323, -26.3711) (54.3027, -26.134) knots 0 0 0 1 2 2 2
  spline S136 degree 2 poles (54.3027, -26.134) (54.4682, -25.9018) (54.9919, -25.6425) (55.3352, -25.6425) knots 0 0 0 1 2 2 2
  spline S137 degree 2 poles (55.3352, -25.6425) (55.4365, -25.6425) (55.6143, -25.6622) (55.681, -25.6845) knots 0 0 0 1 2 2 2
  line L198 (55.681, -25.6845) -> (55.681, -26.0772)
  line L199 (55.681, -26.0772) -> (55.6637, -26.0772)
  spline S138 degree 2 poles (55.6637, -26.0772) (55.6069, -26.0476) (55.3994, -25.9957) (55.2809, -25.9957) knots 0 0 0 1 2 2 2
  spline S139 degree 2 poles (55.2809, -25.9957) (54.9005, -25.9957) (54.4337, -26.5095) (54.3892, -27.0133) knots 0 0 0 1 2 2 2
  spline S140 degree 2 poles (54.3892, -27.0133) (54.5349, -26.9121) (54.8412, -26.8009) (55.024, -26.8009) knots 0 0 0 1 2 2 2
  spline S141 degree 2 poles (55.024, -26.8009) (55.2018, -26.8009) (55.4686, -26.8725) (55.6143, -26.9812) knots 0 0 0 1 2 2 2
  spline S142 degree 2 poles (55.6143, -26.9812) (55.7823, -27.1072) (55.9453, -27.4975) (55.9453, -27.7593) knots 0 0 0 1 2 2 2
  spline S143 degree 2 poles (55.5303, -27.7766) (55.5303, -27.5889) (55.4315, -27.3344) (55.3229, -27.2455) knots 0 0 0 1 2 2 2
  spline S144 degree 2 poles (55.3229, -27.2455) (55.2414, -27.1813) (55.0388, -27.1393) (54.9326, -27.1393) knots 0 0 0 1 2 2 2
  spline S145 degree 2 poles (54.9326, -27.1393) (54.7893, -27.1393) (54.5201, -27.2258) (54.3892, -27.3073) knots 0 0 0 1 2 2 2
  spline S146 degree 2 poles (54.3892, -27.3073) (54.3867, -27.3517) (54.3818, -27.4357) (54.3818, -27.4999) knots 0 0 0 1 2 2 2
  spline S147 degree 2 poles (54.3818, -27.4999) (54.3818, -27.8161) (54.5053, -28.2039) (54.5992, -28.3052) knots 0 0 0 1 2 2 2
  spline S148 degree 2 poles (54.5992, -28.3052) (54.6856, -28.4015) (54.8733, -28.4781) (54.9795, -28.4781) knots 0 0 0 1 2 2 2
  spline S149 degree 2 poles (54.9795, -28.4781) (55.2265, -28.4781) (55.5303, -28.1273) (55.5303, -27.7766) knots 0 0 0 1 2 2 2
  spline S150 degree 2 poles (57.1284, -25.9883) (57.0173, -25.9883) (56.7975, -26.0426) (56.6913, -26.0846) knots 0 0 0 1 2 2 2
  spline S151 degree 2 poles (56.6913, -26.0846) (56.5925, -26.1266) (56.4467, -26.2155) (56.3899, -26.255) knots 0 0 0 1 2 2 2
  line L200 (56.3899, -26.255) -> (56.3652, -26.255)
  line L201 (56.3652, -26.255) -> (56.3652, -25.8228)
  spline S152 degree 2 poles (56.3652, -25.8228) (56.4986, -25.7512) (56.9555, -25.6351) (57.1606, -25.6351) knots 0 0 0 1 2 2 2
  spline S153 degree 2 poles (57.1606, -25.6351) (57.368, -25.6351) (57.6768, -25.7191) (57.8028, -25.808) knots 0 0 0 1 2 2 2
  spline S154 degree 2 poles (57.8028, -25.808) (57.9361, -25.9043) (58.0745, -26.1834) (58.0745, -26.3711) knots 0 0 0 1 2 2 2
  spline S155 degree 2 poles (58.0745, -26.3711) (58.0745, -26.6231) (57.7435, -27.0035) (57.5113, -27.0529) knots 0 0 0 1 2 2 2
  line L202 (57.5113, -27.0529) -> (57.5113, -27.0825)
  spline S156 degree 2 poles (57.5113, -27.0825) (57.6076, -27.1023) (57.8275, -27.1912) (57.9213, -27.2801) knots 0 0 0 1 2 2 2
  spline S157 degree 2 poles (57.9213, -27.2801) (58.0152, -27.3666) (58.1337, -27.6432) (58.1337, -27.8433) knots 0 0 0 1 2 2 2
  spline S158 degree 2 poles (58.1337, -27.8433) (58.1337, -28.0483) (57.993, -28.3965) (57.8645, -28.5299) knots 0 0 0 1 2 2 2
  spline S159 degree 2 poles (57.8645, -28.5299) (57.7311, -28.6683) (57.3532, -28.8115) (57.1136, -28.8115) knots 0 0 0 1 2 2 2
  spline S160 degree 2 poles (57.1136, -28.8115) (56.8839, -28.8115) (56.4344, -28.7004) (56.2812, -28.6238) knots 0 0 0 1 2 2 2
  line L203 (56.2812, -28.6238) -> (56.2812, -28.1915)
  line L204 (56.2812, -28.1915) -> (56.3109, -28.1915)
  spline S161 degree 2 poles (56.3109, -28.1915) (56.4393, -28.2854) (56.874, -28.4583) (57.0889, -28.4583) knots 0 0 0 1 2 2 2
  spline S162 degree 2 poles (57.0889, -28.4583) (57.2149, -28.4583) (57.4668, -28.3793) (57.5508, -28.2879) knots 0 0 0 1 2 2 2
  spline S163 degree 2 poles (57.5508, -28.2879) (57.6323, -28.1965) (57.7188, -27.9791) (57.7188, -27.8136) knots 0 0 0 1 2 2 2
  spline S164 degree 2 poles (57.7188, -27.8136) (57.7188, -27.6481) (57.6225, -27.4332) (57.536, -27.3715) knots 0 0 0 1 2 2 2
  spline S165 degree 2 poles (57.536, -27.3715) (57.4495, -27.3097) (57.2149, -27.2628) (57.0766, -27.2628) knots 0 0 0 1 2 2 2
  line L205 (57.0766, -27.2628) -> (56.9037, -27.2628)
  line L206 (56.9037, -27.2628) -> (56.9037, -26.9244)
  line L207 (56.9037, -26.9244) -> (57.0395, -26.9244)
  spline S166 degree 2 poles (57.0395, -26.9244) (57.3137, -26.9244) (57.6595, -26.6626) (57.6595, -26.4131) knots 0 0 0 1 2 2 2
  spline S167 degree 2 poles (57.6595, -26.4131) (57.6595, -26.297) (57.5706, -26.1315) (57.4989, -26.0821) knots 0 0 0 1 2 2 2
  spline S168 degree 2 poles (57.4989, -26.0821) (57.4224, -26.0303) (57.2347, -25.9883) (57.1284, -25.9883) knots 0 0 0 1 2 2 2
  spline S169 degree 2 poles (60.5198, -27.7593) (60.5198, -27.9939) (60.3642, -28.3916) (60.2333, -28.525) knots 0 0 0 1 2 2 2
  spline S170 degree 2 poles (60.2333, -28.525) (60.0974, -28.6658) (59.7565, -28.8115) (59.5515, -28.8115) knots 0 0 0 1 2 2 2
  spline S171 degree 2 poles (59.5515, -28.8115) (59.3465, -28.8115) (59.0081, -28.6732) (58.8797, -28.5349) knots 0 0 0 1 2 2 2
  spline S172 degree 2 poles (58.8797, -28.5349) (58.7216, -28.3694) (58.5438, -27.8136) (58.5438, -27.4085) knots 0 0 0 1 2 2 2
  spline S173 degree 2 poles (58.5438, -27.4085) (58.5438, -27.0109) (58.7068, -26.3711) (58.8772, -26.134) knots 0 0 0 1 2 2 2
  spline S174 degree 2 poles (58.8772, -26.134) (59.0427, -25.9018) (59.5664, -25.6425) (59.9097, -25.6425) knots 0 0 0 1 2 2 2
  spline S175 degree 2 poles (59.9097, -25.6425) (60.011, -25.6425) (60.1888, -25.6622) (60.2555, -25.6845) knots 0 0 0 1 2 2 2
  line L208 (60.2555, -25.6845) -> (60.2555, -26.0772)
  line L209 (60.2555, -26.0772) -> (60.2382, -26.0772)
  spline S176 degree 2 poles (60.2382, -26.0772) (60.1814, -26.0476) (59.9739, -25.9957) (59.8553, -25.9957) knots 0 0 0 1 2 2 2
  spline S177 degree 2 poles (59.8553, -25.9957) (59.475, -25.9957) (59.0081, -26.5095) (58.9637, -27.0133) knots 0 0 0 1 2 2 2
  spline S178 degree 2 poles (58.9637, -27.0133) (59.1094, -26.9121) (59.4157, -26.8009) (59.5985, -26.8009) knots 0 0 0 1 2 2 2
  spline S179 degree 2 poles (59.5985, -26.8009) (59.7763, -26.8009) (60.0431, -26.8725) (60.1888, -26.9812) knots 0 0 0 1 2 2 2
  spline S180 degree 2 poles (60.1888, -26.9812) (60.3568, -27.1072) (60.5198, -27.4975) (60.5198, -27.7593) knots 0 0 0 1 2 2 2
  spline S181 degree 2 poles (60.1048, -27.7766) (60.1048, -27.5889) (60.006, -27.3344) (59.8973, -27.2455) knots 0 0 0 1 2 2 2
  spline S182 degree 2 poles (59.8973, -27.2455) (59.8158, -27.1813) (59.6133, -27.1393) (59.5071, -27.1393) knots 0 0 0 1 2 2 2
  spline S183 degree 2 poles (59.5071, -27.1393) (59.3638, -27.1393) (59.0946, -27.2258) (58.9637, -27.3073) knots 0 0 0 1 2 2 2
  spline S184 degree 2 poles (58.9637, -27.3073) (58.9612, -27.3517) (58.9563, -27.4357) (58.9563, -27.4999) knots 0 0 0 1 2 2 2
  spline S185 degree 2 poles (58.9563, -27.4999) (58.9563, -27.8161) (59.0798, -28.2039) (59.1736, -28.3052) knots 0 0 0 1 2 2 2
  spline S186 degree 2 poles (59.1736, -28.3052) (59.2601, -28.4015) (59.4478, -28.4781) (59.554, -28.4781) knots 0 0 0 1 2 2 2
  spline S187 degree 2 poles (59.554, -28.4781) (59.801, -28.4781) (60.1048, -28.1273) (60.1048, -27.7766) knots 0 0 0 1 2 2 2
  spline S188 degree 2 poles (62.7774, -27.2233) (62.7774, -28.0433) (62.3007, -28.8115) (61.8042, -28.8115) knots 0 0 0 1 2 2 2
  spline S189 degree 2 poles (61.8042, -28.8115) (61.3003, -28.8115) (60.8285, -28.0285) (60.8285, -27.2258) knots 0 0 0 1 2 2 2
  spline S190 degree 2 poles (60.8285, -27.2258) (60.8285, -26.4008) (61.3052, -25.6375) (61.8042, -25.6375) knots 0 0 0 1 2 2 2
  spline S191 degree 2 poles (61.8042, -25.6375) (62.3056, -25.6375) (62.7774, -26.4279) (62.7774, -27.2233) knots 0 0 0 1 2 2 2
  spline S192 degree 2 poles (62.2537, -28.152) (62.313, -28.0013) (62.3624, -27.537) (62.3624, -27.2233) knots 0 0 0 1 2 2 2
  spline S193 degree 2 poles (62.3624, -27.2233) (62.3624, -26.9096) (62.313, -26.4477) (62.2513, -26.2921) knots 0 0 0 1 2 2 2
  spline S194 degree 2 poles (62.2513, -26.2921) (62.1895, -26.1365) (61.9746, -25.9759) (61.8042, -25.9759) knots 0 0 0 1 2 2 2
  spline S195 degree 2 poles (61.8042, -25.9759) (61.6338, -25.9759) (61.4139, -26.1365) (61.3497, -26.297) knots 0 0 0 1 2 2 2
  spline S196 degree 2 poles (61.3497, -26.297) (61.288, -26.4526) (61.2435, -26.9269) (61.2435, -27.2258) knots 0 0 0 1 2 2 2
  spline S197 degree 2 poles (61.2435, -27.2258) (61.2435, -27.5469) (61.283, -27.9766) (61.3472, -28.1446) knots 0 0 0 1 2 2 2
  spline S198 degree 2 poles (61.3472, -28.1446) (61.4065, -28.3027) (61.6263, -28.4731) (61.8042, -28.4731) knots 0 0 0 1 2 2 2
  spline S199 degree 2 poles (61.8042, -28.4731) (61.9721, -28.4731) (62.192, -28.3126) (62.2537, -28.152) knots 0 0 0 1 2 2 2
  line L210 (65.1288, -27.7) -> (64.7657, -27.7)
  line L211 (64.7657, -27.7) -> (64.7657, -28.7473)
  line L212 (64.7657, -28.7473) -> (64.373, -28.7473)
  line L213 (64.373, -28.7473) -> (64.373, -27.7)
  line L214 (64.373, -27.7) -> (63.0268, -27.7)
  line L215 (63.0268, -27.7) -> (63.0268, -27.2702)
  line L216 (63.0268, -27.2702) -> (64.3903, -25.6993)
  line L217 (64.3903, -25.6993) -> (64.7657, -25.6993)
  line L218 (64.7657, -25.6993) -> (64.7657, -27.3715)
  line L219 (64.7657, -27.3715) -> (65.1288, -27.3715)
  line L220 (65.1288, -27.3715) -> (65.1288, -27.7)
  line L221 (64.373, -27.3715) -> (64.373, -26.1809)
  line L222 (64.373, -26.1809) -> (63.3479, -27.3715)
  line L223 (63.3479, -27.3715) -> (64.373, -27.3715)
  point P0 (0, 0)
  constraints: 4 other
extrude "PhoneNumber" cut sketch "Sketch24" against normal blind 0.5
sketch "Sketch25" plane through (0, 0, 0) normal (0, -1, 0) x (1, 0, 0)
  line L0 (61.0662, 20.9281) -> (73.8693, 20.9281) construction
  line L1 (73.8693, 20.9281) -> (73.8693, 15.5184) construction
  line L2 (73.8693, 15.5184) -> (61.0662, 15.5184) construction
  line L3 (61.0662, 15.5184) -> (61.0662, 20.9281) construction
  line L4 (63.224, 20.0727) -> (62.3275, 17.6939)
  line L5 (62.3275, 17.6939) -> (61.9679, 17.6939)
  line L6 (61.9679, 17.6939) -> (61.079, 20.0727)
  line L7 (61.079, 20.0727) -> (61.5132, 20.0727)
  line L8 (61.5132, 20.0727) -> (62.1631, 18.2411)
  line L9 (62.1631, 18.2411) -> (62.8079, 20.0727)
  line L10 (62.8079, 20.0727) -> (63.224, 20.0727)
  line L11 (65.2637, 17.6939) -> (63.7173, 17.6939)
  line L12 (63.7173, 17.6939) -> (63.7173, 18.0176)
  line L13 (63.7173, 18.0176) -> (64.2927, 18.0176)
  line L14 (64.2927, 18.0176) -> (64.2927, 20.1421)
  line L15 (64.2927, 20.1421) -> (63.7173, 20.1421)
  line L16 (63.7173, 20.1421) -> (63.7173, 20.4324)
  spline S0 degree 2 poles (63.7173, 20.4324) (64.0435, 20.4324) (64.3518, 20.6173) (64.3723, 20.8742) knots 0 0 0 1 2 2 2
  line L17 (64.3723, 20.8742) -> (64.7011, 20.8742)
  line L18 (64.7011, 20.8742) -> (64.7011, 18.0176)
  line L19 (64.7011, 18.0176) -> (65.2637, 18.0176)
  line L20 (65.2637, 18.0176) -> (65.2637, 17.6939)
  line L21 (66.5276, 17.6939) -> (66.019, 17.6939)
  line L22 (66.019, 17.6939) -> (66.019, 18.3002)
  line L23 (66.019, 18.3002) -> (66.5276, 18.3002)
  line L24 (66.5276, 18.3002) -> (66.5276, 17.6939)
  spline S1 degree 2 poles (69.1402, 19.2789) (69.1402, 18.4261) (68.6444, 17.6271) (68.128, 17.6271) knots 0 0 0 1 2 2 2
  spline S2 degree 2 poles (68.128, 17.6271) (67.604, 17.6271) (67.1133, 18.4415) (67.1133, 19.2764) knots 0 0 0 1 2 2 2
  spline S3 degree 2 poles (67.1133, 19.2764) (67.1133, 20.1344) (67.6091, 20.9281) (68.128, 20.9281) knots 0 0 0 1 2 2 2
  spline S4 degree 2 poles (68.128, 20.9281) (68.6495, 20.9281) (69.1402, 20.1061) (69.1402, 19.2789) knots 0 0 0 1 2 2 2
  spline S5 degree 2 poles (68.5956, 18.313) (68.6572, 18.4697) (68.7086, 18.9527) (68.7086, 19.2789) knots 0 0 0 1 2 2 2
  spline S6 degree 2 poles (68.7086, 19.2789) (68.7086, 19.6052) (68.6572, 20.0856) (68.593, 20.2474) knots 0 0 0 1 2 2 2
  spline S7 degree 2 poles (68.593, 20.2474) (68.5288, 20.4092) (68.3053, 20.5762) (68.128, 20.5762) knots 0 0 0 1 2 2 2
  spline S8 degree 2 poles (68.128, 20.5762) (67.9508, 20.5762) (67.7221, 20.4092) (67.6554, 20.2423) knots 0 0 0 1 2 2 2
  spline S9 degree 2 poles (67.6554, 20.2423) (67.5911, 20.0804) (67.5449, 19.5872) (67.5449, 19.2764) knots 0 0 0 1 2 2 2
  spline S10 degree 2 poles (67.5449, 19.2764) (67.5449, 18.9424) (67.586, 18.4954) (67.6528, 18.3207) knots 0 0 0 1 2 2 2
  spline S11 degree 2 poles (67.6528, 18.3207) (67.7144, 18.1563) (67.9431, 17.9791) (68.128, 17.9791) knots 0 0 0 1 2 2 2
  spline S12 degree 2 poles (68.128, 17.9791) (68.3027, 17.9791) (68.5313, 18.146) (68.5956, 18.313) knots 0 0 0 1 2 2 2
  line L25 (70.2268, 17.6939) -> (69.7182, 17.6939)
  line L26 (69.7182, 17.6939) -> (69.7182, 18.3002)
  line L27 (69.7182, 18.3002) -> (70.2268, 18.3002)
  line L28 (70.2268, 18.3002) -> (70.2268, 17.6939)
  line L29 (72.6621, 17.6939) -> (71.1156, 17.6939)
  line L30 (71.1156, 17.6939) -> (71.1156, 18.0176)
  line L31 (71.1156, 18.0176) -> (71.6911, 18.0176)
  line L32 (71.6911, 18.0176) -> (71.6911, 20.1421)
  line L33 (71.6911, 20.1421) -> (71.1156, 20.1421)
  line L34 (71.1156, 20.1421) -> (71.1156, 20.4324)
  spline S13 degree 2 poles (71.1156, 20.4324) (71.4419, 20.4324) (71.7502, 20.6173) (71.7707, 20.8742) knots 0 0 0 1 2 2 2
  line L35 (71.7707, 20.8742) -> (72.0995, 20.8742)
  line L36 (72.0995, 20.8742) -> (72.0995, 18.0176)
  line L37 (72.0995, 18.0176) -> (72.6621, 18.0176)
  line L38 (72.6621, 18.0176) -> (72.6621, 17.6939)
  point P0 (0, 0)
  constraints: 2 other
extrude "VersionNumber" cut sketch "Sketch25" against normal blind 0.5
body "Solid4"
